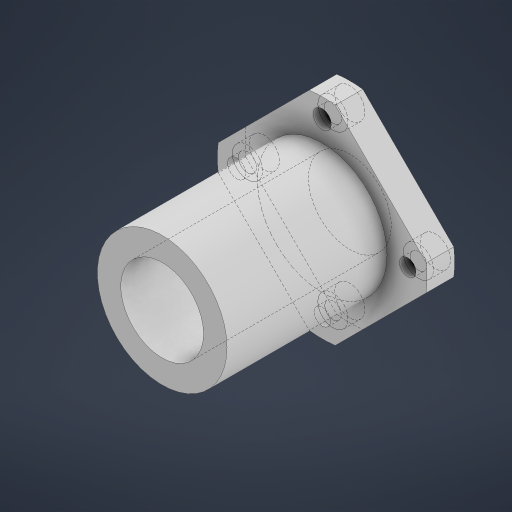
# Autodesk Inventor part: LMEK30UU
Saved by Autodesk Inventor 2023 (Build 270158000, 158)
## iProperties
Created: 2025-09-03
Part Number: LMEK30UU
Material: 일반
Document SubType Name: Modeling
Designer: k
Density: 1 g/cm^3
Appearance: 기본값
Author: k
Autodesk Inventor part; units mm, degrees
ref_plane "YZ Plane" through (0, 0, 0) normal (1, 0, 0) x (0, 1, 0)
ref_plane "XZ Plane" through (0, 0, 0) normal (0, 1, 0) x (-1, 0, 0)
ref_plane "XY Plane" through (0, 0, 0) normal (0, 0, 1) x (1, 0, 0)
sketch "스케치1" plane through (0, 0, 0) normal (0, 0, 1) x (1, 0, 0)
  line L0 (105.4763, -137.5312) -> (138.4611, -104.5464)
  arc A0 (147.9027, -104.5464) -> (138.4611, -104.5464) centre (143.1819, -142.252) ccw
  arc A1 (105.4763, -137.5312) -> (105.4763, -146.9728) centre (143.1819, -142.252) ccw
  line L1 (105.4763, -146.9728) -> (138.4611, -179.9576)
  arc A2 (138.4611, -179.9576) -> (147.9027, -179.9576) centre (143.1819, -142.252) ccw
  arc A3 (180.8875, -146.9728) -> (180.8875, -137.5312) centre (143.1819, -142.252) ccw
  line L2 (147.9027, -179.9576) -> (180.8875, -146.9728)
  line L3 (147.9027, -104.5464) -> (180.8875, -137.5312)
  circle A4 centre (143.1819, -142.252) radius 31
  circle A5 centre (143.1819, -111.252) radius 3.3
  circle A6 centre (174.1819, -142.252) radius 3
  circle A7 centre (143.1819, -173.252) radius 3
  circle A8 centre (112.1819, -142.252) radius 3.3
  dimension "d13" = 38
  dimension "d14" = 38
  dimension "d15" = 38
  dimension "d16" = 38
  dimension "d17" = 60
  dimension "d18" = 60
  dimension "d19" = 62
  dimension "d20" = 6.6
  dimension "d21" = 6
  dimension "d22" = 6
  dimension "d23" = 6.6
  constraints: 12 point on circle, 9 centre point, 8 end point, 1 coincident
  measures "d13" radius of A0
  measures "d14" radius of A3
  measures "d15" radius of A2
  measures "d16" radius of A1
  measures "d17" distance between parallel lines of L1 L3
  measures "d18" distance between parallel lines of L2 L0
  measures "d19" diameter of A4
  measures "d20" diameter of A5
  measures "d21" diameter of A6
  measures "d22" diameter of A7
  measures "d23" diameter of A8
extrude "돌출1" add sketch "스케치1" along normal blind 10 contours L0 A4 A8 L1 A1 | L0 A4 A5 L3 A6 L2 A7 L1 A8 | L0 A0 L3 A4 A5 | A4 A7 L2 A2 L1 | L3 A3 L2 A4 A6
sketch "스케치2" plane through (0, 0, 10) normal (0, 0, 1) x (1, 0, 0)
  arc A0 (147.9027, -104.5464) -> (138.4611, -104.5464) centre (143.1819, -142.252) ccw projected
  circle A1 centre (143.1819, -142.252) radius 23.5
  dimension "d26" = 47
  constraints: 1 centre point, 1 coincident
  measures "d26" diameter of A1
extrude "돌출2" add sketch "스케치2" along normal blind 58
sketch "스케치3" plane through (143.1819, -142.252, 68) normal (0, 0, 1) x (1, 0, 0)
  circle A0 centre (0, 0) radius 15
  dimension "d29" = 30
  constraints: 1 centre point
  measures "d29" diameter of A0
extrude "돌출3" cut sketch "스케치3" against normal through all
sketch "스케치4" plane through (0, 0, 0) normal (0, 0, -1) x (-1, 0, 0)
  circle A0 centre (-143.1819, -142.252) radius 15 projected
  circle A1 centre (-143.1819, -142.252) radius 31
  circle A2 centre (-143.1819, -111.252) radius 3.3 projected
  circle A3 centre (-143.1819, -111.252) radius 5.5
  circle A4 centre (-174.1819, -142.252) radius 5.5
  circle A5 centre (-143.1819, -173.252) radius 5.5
  circle A6 centre (-112.1819, -142.252) radius 5.5
  dimension "d32" = 62
  dimension "d33" = 11
  dimension "d34" = 11
  dimension "d35" = 11
  dimension "d36" = 11
  constraints: 5 centre point, 3 point on circle, 2 coincident
  measures "d32" diameter of A1
  measures "d33" diameter of A3
  measures "d34" diameter of A4
  measures "d35" diameter of A5
  measures "d36" diameter of A6
extrude "돌출4" cut sketch "스케치4" against normal blind 6.1 contours A1 A6 | A1 A6 | A3 A1 A2 | A1 A2 A3 | A5 A1 | A1 A5 | A2 A1 | A1 A2 | A4 A1 | A1 A4
